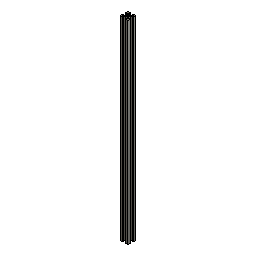
2020 Extrusion v2 (Autodesk Fusion 360 design; units mm, degrees)
Autodesk Fusion 360 part; units mm, degrees
sketch "Sketch1" plane through (0, 0, 503) normal (0, 0, 1) x (1, 0, 0)
  line L0 (2.84, -3.9007) -> (5.4993, -6.56)
  line L1 (5.4993, -6.56) -> (5.4993, -8.2)
  line L2 (5.4993, -8.2) -> (2.84, -8.2)
  line L3 (2.84, -8.2) -> (4.64, -10)
  line L4 (4.64, -10) -> (10, -10)
  line L5 (10, -10) -> (10, -4.64)
  line L6 (10, -4.64) -> (8.2, -2.84)
  line L7 (8.2, -2.84) -> (8.2, -5.4993)
  line L8 (8.2, -5.4993) -> (6.56, -5.4993)
  line L9 (6.56, -5.4993) -> (3.9007, -2.84)
  line L10 (3.9007, -2.84) -> (3.9007, 2.84)
  line L11 (3.9007, 2.84) -> (6.56, 5.4993)
  line L12 (6.56, 5.4993) -> (8.2, 5.4993)
  line L13 (8.2, 5.4993) -> (8.2, 2.84)
  line L14 (8.2, 2.84) -> (10, 4.64)
  line L15 (10, 4.64) -> (10, 10)
  line L16 (10, 10) -> (4.64, 10)
  line L17 (4.64, 10) -> (2.84, 8.2)
  line L18 (2.84, 8.2) -> (5.4993, 8.2)
  line L19 (5.4993, 8.2) -> (5.4993, 6.56)
  line L20 (5.4993, 6.56) -> (2.84, 3.9007)
  line L21 (2.84, 3.9007) -> (-2.84, 3.9007)
  line L22 (-2.84, 3.9007) -> (-5.4993, 6.56)
  line L23 (-5.4993, 6.56) -> (-5.4993, 8.2)
  line L24 (-5.4993, 8.2) -> (-2.84, 8.2)
  line L25 (-2.84, 8.2) -> (-4.64, 10)
  line L26 (-4.64, 10) -> (-10, 10)
  line L27 (-10, 10) -> (-10, 4.64)
  line L28 (-10, 4.64) -> (-8.2, 2.84)
  line L29 (-8.2, 2.84) -> (-8.2, 5.4993)
  line L30 (-8.2, 5.4993) -> (-6.56, 5.4993)
  line L31 (-6.56, 5.4993) -> (-3.9007, 2.84)
  line L32 (-3.9007, 2.84) -> (-3.9007, -2.84)
  line L33 (-3.9007, -2.84) -> (-6.56, -5.4993)
  line L34 (-6.56, -5.4993) -> (-8.2, -5.4993)
  line L35 (-8.2, -5.4993) -> (-8.2, -2.84)
  line L36 (-8.2, -2.84) -> (-10, -4.64)
  line L37 (-10, -4.64) -> (-10, -10)
  line L38 (-10, -10) -> (-4.64, -10)
  line L39 (-4.64, -10) -> (-2.84, -8.2)
  line L40 (-2.84, -8.2) -> (-5.4993, -8.2)
  line L41 (-5.4993, -8.2) -> (-5.4993, -6.56)
  line L42 (-5.4993, -6.56) -> (-2.84, -3.9007)
  line L43 (-2.84, -3.9007) -> (2.84, -3.9007)
  circle A0 centre (0, 0) radius 2.1
  circle A1 centre (0, 0) radius 2.1
  line L44 (-2.84, -3.9007) -> (2.84, -3.9007)
  line L45 (-3.9007, 2.84) -> (-3.9007, -2.84)
  line L46 (2.84, 3.9007) -> (-2.84, 3.9007)
  line L47 (3.9007, -2.84) -> (3.9007, 2.84)
  line L48 (5.4993, 6.56) -> (2.84, 3.9007)
  line L49 (5.4993, 8.2) -> (5.4993, 6.56)
  line L50 (2.84, 8.2) -> (5.4993, 8.2)
  line L51 (4.64, 10) -> (2.84, 8.2)
  line L52 (10, 10) -> (4.64, 10)
  line L53 (10, 4.64) -> (10, 10)
  line L54 (8.2, 2.84) -> (10, 4.64)
  line L55 (8.2, 5.4993) -> (8.2, 2.84)
  line L56 (6.56, 5.4993) -> (8.2, 5.4993)
  line L57 (3.9007, 2.84) -> (6.56, 5.4993)
  line L58 (-5.4993, -6.56) -> (-2.84, -3.9007)
  line L59 (-5.4993, -8.2) -> (-5.4993, -6.56)
  line L60 (-2.84, -8.2) -> (-5.4993, -8.2)
  line L61 (-4.64, -10) -> (-2.84, -8.2)
  line L62 (-10, -10) -> (-4.64, -10)
  line L63 (-10, -4.64) -> (-10, -10)
  line L64 (-8.2, -2.84) -> (-10, -4.64)
  line L65 (-8.2, -5.4993) -> (-8.2, -2.84)
  line L66 (-6.56, -5.4993) -> (-8.2, -5.4993)
  line L67 (-3.9007, -2.84) -> (-6.56, -5.4993)
  line L68 (-6.56, 5.4993) -> (-3.9007, 2.84)
  line L69 (-8.2, 5.4993) -> (-6.56, 5.4993)
  line L70 (-8.2, 2.84) -> (-8.2, 5.4993)
  line L71 (-10, 4.64) -> (-8.2, 2.84)
  line L72 (-10, 10) -> (-10, 4.64)
  line L73 (-4.64, 10) -> (-10, 10)
  line L74 (-2.84, 8.2) -> (-4.64, 10)
  line L75 (-5.4993, 8.2) -> (-2.84, 8.2)
  line L76 (-5.4993, 6.56) -> (-5.4993, 8.2)
  line L77 (-2.84, 3.9007) -> (-5.4993, 6.56)
  line L78 (6.56, -5.4993) -> (3.9007, -2.84)
  line L79 (8.2, -5.4993) -> (6.56, -5.4993)
  line L80 (8.2, -2.84) -> (8.2, -5.4993)
  line L81 (10, -4.64) -> (8.2, -2.84)
  line L82 (10, -10) -> (10, -4.64)
  line L83 (4.64, -10) -> (10, -10)
  line L84 (2.84, -8.2) -> (4.64, -10)
  line L85 (5.4993, -8.2) -> (2.84, -8.2)
  line L86 (5.4993, -6.56) -> (5.4993, -8.2)
  line L87 (2.84, -3.9007) -> (5.4993, -6.56)
extrude "Extrude1" add sketch "Sketch1" along normal blind 489 makes body 1
copy_body "Body->Comp1" bodies 1 removing the originals makes body 2 in component "489mm 2020"
component "489mm 2020" placed x (1, 0, 0) y (0, 1, 0) z (0, 0, 1) at (0, 0, 0)
named bodies: "489mm 2020"
